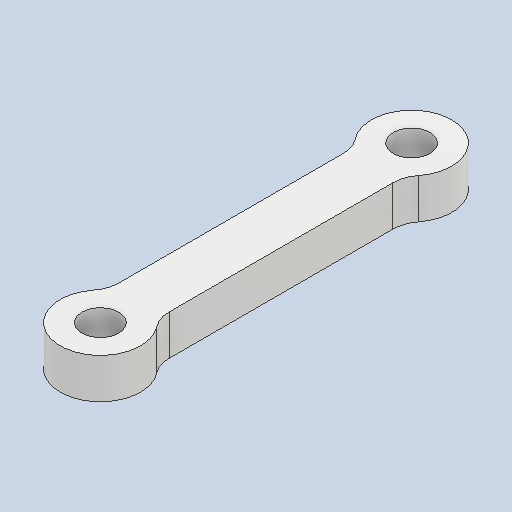
# Autodesk Inventor part: spojka
Saved by Autodesk Inventor 2023 (Build 270158000, 158)
## iProperties
Part Number: spojka
Material: ABS Plastic
Document SubType Name: Modeling
Designer: denyh
Density: 1.06 g/cm^3
Appearance: Smooth - White
Mass: 0.8396 g
Surface Area: 8.41719 cm^2
Volume: 0.792076 cm^3
Author: denyh
Autodesk Inventor part; units mm, degrees
ref_plane "YZ Plane" through (0, 0, 0) normal (1, 0, 0) x (0, 1, 0)
ref_plane "XZ Plane" through (0, 0, 0) normal (0, 1, 0) x (-1, 0, 0)
ref_plane "XY Plane" through (0, 0, 0) normal (0, 0, 1) x (1, 0, 0)
sketch "Náčrt1" plane through (0, 0, 0) normal (0, 0, 1) x (1, 0, 0)
  line L0 (0, 0) -> (0, 31)
  circle A0 centre (0, 31) radius 1.825
  circle A1 centre (0, 0) radius 1.825
  arc A2 (3.1429, 28.5257) -> (-3.1429, 28.5257) centre (0, 31) ccw
  arc A3 (-3.1429, 2.4743) -> (3.1429, 2.4743) centre (0, 0) ccw
  line L1 (0, 31) -> (-5.5, 31)
  line L2 (-5.5, 31) -> (-5.5, 26.67)
  arc A4 (-2.5003, 26.6349) -> (-3.1429, 28.5257) centre (-5.5, 26.67) ccw
  line L3 (-2.5003, 4.2949) -> (-2.5003, 15.5)
  arc A5 (3.1429, 28.5257) -> (2.5003, 26.6349) centre (5.5, 26.67) ccw
  arc A6 (-3.1429, 2.4743) -> (-2.5003, 4.3651) centre (-5.5, 4.33) ccw
  arc A7 (2.5003, 4.3651) -> (3.1429, 2.4743) centre (5.5, 4.33) ccw
  line L4 (2.5003, 26.6349) -> (2.5003, 4.3651)
  line L5 (-2.5003, 26.6349) -> (-2.5003, 15.5)
  dimension "d0" = 31
  dimension "d1" = 3.65
  dimension "d2" = 3.65
  dimension "d3" = 8
  dimension "d4" = 8
  dimension "d7" = 5.5
  dimension "d8" = 4.33
  constraints: 13 point on circle, 12 end point, 8 centre point, 5 coincident, 3 symmetric about line, 3 vertical, 1 collinear, 1 horizontal, 1 parallel, 1 point on line, 1 tangent, 1 other
  measures "d0" distance of L0.start L0.end
  measures "d1" diameter of A0
  measures "d2" diameter of A1
  measures "d3" diameter of A2
  measures "d4" diameter of A3
  measures "d7" distance of L1.start L1.end
  measures "d8" distance of L1.end L2.end
extrude "Vysunutí1" add sketch "Náčrt1" along normal blind 4
